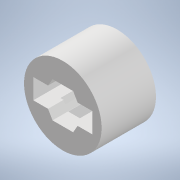
# Autodesk Inventor part: mixer_gear
Saved by Autodesk Inventor 2022 (Build 260153000, 153)
## iProperties
Created: 2022-06-21
Part Number: mixer_gear
Material: Generic
Document SubType Name: Modeling
Designer: efred
Density: 1 g/cm^3
Appearance: Default
Author: efred
Autodesk Inventor part; units mm, degrees
ref_plane "YZ Plane" through (0, 0, 0) normal (1, 0, 0) x (0, 1, 0)
ref_plane "XZ Plane" through (0, 0, 0) normal (0, 1, 0) x (-1, 0, 0)
ref_plane "XY Plane" through (0, 0, 0) normal (0, 0, 1) x (1, 0, 0)
sketch "Sketch1" plane through (0, 0, 0) normal (0, 0, 1) x (1, 0, 0)
  circle A0 centre (0, 0) radius 0.5 projected
  line L0 (-1.1547, -2) -> (-1.7321, -1) projected
  line L1 (-1.7321, -1) -> (-3.5, -1) projected
  line L2 (-3.5, -1) -> (-3.5, 1) projected
  line L3 (-3.5, 1) -> (-1.7321, 1) projected
  line L4 (-1.7321, 1) -> (-1.1547, 2) projected
  line L5 (-1.1547, 2) -> (1.1547, 2) projected
  line L6 (1.1547, 2) -> (1.7321, 1) projected
  line L7 (1.7321, 1) -> (3.5, 1) projected
  line L8 (3.5, 1) -> (3.5, -1) projected
  line L9 (3.5, -1) -> (1.7321, -1) projected
  line L10 (1.7321, -1) -> (1.1547, -2) projected
  line L11 (1.1547, -2) -> (-1.1547, -2) projected
  circle A1 centre (0, 0) radius 5
  line L12 (-3.8, -1.3) -> (-1.9053, -1.3)
  line L13 (-1.9053, -1.3) -> (-1.3279, -2.3)
  line L14 (-1.3279, -2.3) -> (1.3279, -2.3)
  line L15 (1.3279, -2.3) -> (1.9053, -1.3)
  line L16 (1.9053, -1.3) -> (3.8, -1.3)
  line L17 (3.8, -1.3) -> (3.8, 1.3)
  line L18 (3.8, 1.3) -> (1.9053, 1.3)
  line L19 (1.9053, 1.3) -> (1.3279, 2.3)
  line L20 (1.3279, 2.3) -> (-1.3279, 2.3)
  line L21 (-1.3279, 2.3) -> (-1.9053, 1.3)
  line L22 (-1.9053, 1.3) -> (-3.8, 1.3)
  line L23 (-3.8, 1.3) -> (-3.8, -1.3)
  dimension "d0" = 10
  dimension "d1" = 0.3
  constraints: 24 end point, 1 centre point, 1 coincident, 11 other
  measures "d0" diameter of A1
  measures "d1" distance between parallel lines of L1 L12
extrude "Extrusion1" add sketch "Sketch1" along normal blind 2 and the other way blind 5 contours A1
sketch "Sketch2" plane through (0, 0, -5) normal (0, 0, -1) x (-1, 0, 0)
  circle A0 centre (0, 0) radius 5 projected
  line L0 (3.8, 1.3) -> (3.8, -1.3) projected
  line L1 (3.8, -1.3) -> (1.9053, -1.3) projected
  line L2 (1.9053, -1.3) -> (1.3279, -2.3) projected
  line L3 (1.3279, -2.3) -> (-1.3279, -2.3) projected
  line L4 (-1.3279, -2.3) -> (-1.9053, -1.3) projected
  line L5 (-1.9053, -1.3) -> (-3.8, -1.3) projected
  line L6 (-3.8, -1.3) -> (-3.8, 1.3) projected
  line L7 (-3.8, 1.3) -> (-1.9053, 1.3) projected
  line L8 (-1.9053, 1.3) -> (-1.3279, 2.3) projected
  line L9 (-1.3279, 2.3) -> (1.3279, 2.3) projected
  line L10 (1.3279, 2.3) -> (1.9053, 1.3) projected
  line L11 (1.9053, 1.3) -> (3.8, 1.3) projected
  line L12 (3.8, 1.3) -> (3.8, -1.3) projected
  line L13 (3.8, 1.3) -> (3.8, -1.3)
  line L14 (3.8, -1.3) -> (1.9053, -1.3)
  line L15 (1.9053, -1.3) -> (1.3279, -2.3) projected
  line L16 (1.9053, -1.3) -> (1.3279, -2.3)
  line L17 (-1.9053, -1.3) -> (-1.3279, -2.3) projected
  line L18 (-1.3279, -2.3) -> (1.3279, -2.3)
  line L19 (1.9053, 1.3) -> (3.8, 1.3) projected
  line L20 (3.8, 1.3) -> (1.9053, 1.3)
  line L21 (1.3279, 2.3) -> (1.9053, 1.3) projected
  line L22 (1.9053, 1.3) -> (1.3279, 2.3)
  line L23 (1.3279, 2.3) -> (-1.3279, 2.3)
  line L24 (-1.3, 1.9053) -> (-2.3, 1.3279)
  line L25 (-2.3, 1.3279) -> (-2.3, -1.3279)
  line L26 (2.3, -1.3279) -> (2.3, 1.3279)
  line L27 (1.3, 1.9053) -> (2.3, 1.3279)
  line L28 (1.3, 3.8) -> (1.3, 1.9053)
  line L29 (-1.3, 3.8) -> (-1.3, 1.9053)
  line L30 (-1.3, 3.8) -> (1.3, 3.8)
  line L31 (-1.9053, -1.3) -> (-1.3279, -2.3)
  line L32 (-1.3279, -2.3) -> (1.3279, -2.3)
  line L33 (1.3279, 2.3) -> (-1.3279, 2.3)
  line L34 (-1.9053, 1.3) -> (-1.3279, 2.3)
  line L35 (-3.8, 1.3) -> (-1.9053, 1.3)
  line L36 (-3.8, -1.3) -> (-1.9053, -1.3)
  line L37 (-3.8, -1.3) -> (-3.8, 1.3)
  line L38 (1.3, -1.9053) -> (2.3, -1.3279)
  line L39 (2.3, -1.3279) -> (2.3, 1.3279)
  line L40 (-2.3, 1.3279) -> (-2.3, -1.3279)
  line L41 (-1.3, -1.9053) -> (-2.3, -1.3279)
  line L42 (-1.3, -3.8) -> (-1.3, -1.9053)
  line L43 (1.3, -3.8) -> (1.3, -1.9053)
  line L44 (1.3, -3.8) -> (-1.3, -3.8)
  point P0 (1.3, -2.3)
  point P1 (-1.3, -2.3)
  point P2 (-1.3, 2.3)
  point P3 (1.3, 2.3)
  point P4 (-2.3, 1.3)
  point P5 (-1.6837, 1.6837)
  point P6 (-1.6837, -1.6837)
  point P7 (-2.3, -1.3)
  point P8 (1.6837, -1.6837)
  point P9 (2.3, -1.3)
  point P10 (1.6837, 1.6837)
  point P11 (2.3, 1.3)
  dimension "d8" = 360
  constraints: 56 end point, 4 collinear, 1 point on line, 65 other
ref_plane "Work Plane1" through (-8.8, -2.2, 0) normal (0, 0, 1) x (1, 0, 0)
extrude "Extrusion2" cut sketch "Sketch2" against normal up to surface (5 mm away) contours L11 L10 L27 L26 | L26 L38 L2 L1 | L9 L29 L30 L28 | L43 L44 L42 L3 | L8 L7 L25 L24 | L41 L25 L5 L4
sketch "Sketch3" plane through (0, 0, -5) normal (0, 0, -1) x (-1, 0, 0)
  line L0 (-1.6837, 1.6837) -> (-2.3, 1.3279) projected
  circle A0 centre (0, 0) radius 2.6558
  constraints: 1 coincident, 3 other
extrude "Extrusion3" cut sketch "Sketch3" against normal through all
body "Solid1"
